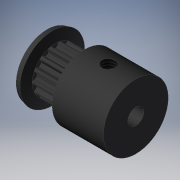
# Autodesk Inventor part: HTPB14S2M040-K-P3_a
Saved by Autodesk Inventor 2019 (Build 230136000, 136)
## iProperties
Created: 2023-12-23
Part Number: HTPB14S2M040-K-P3_a
Material: Generic
Catalog Web Link: www.cadenas.de
Description: HTPA_ _S2M040, HTPA_ _S2M060, HTPA_ _S2M100, HTPB_ _S2M040, HTPB_ _S2M060, HTPB_ _S2M100, HTPK_ _S2M040, HTPK_ _S2M060, HTPK_ _S2M100, HTPN_ _S2M040, HTPN_ _S2M060, HTPN_ _S2M100, HTPT_ _S2M040, HTPT_ _S2M060, HTPM_ _S2M040, HTPM_ _S2M060, HTPP_ _S2M040, HTPP_ _S2M060, HTPS_ _S2M040, HTPS_ _S2M060, HTPS_ _S2M100_a-High Torque Timing Pulleys S2M Type
Vendor: MISUMI
Document SubType Name: Modeling
Designer: psAdmin
Manufacturer: MISUMI
Mass: 1.31576 g
Surface Area: 11.5527 cm^2
Volume: 1.31576 cm^3
Density: 1 g/cm^3
Appearance: PSOLRGB-175-175-175
Category: PARTsolutions
Company: MISUMI
Title: HTPB14S2M040-K-P3
Author: Cadenas PARTsolutions
Comments: High Torque Timing Pulleys S2M Type
PSOL_IDENT_0: {$CADENAS_DATA/23d-libs/misumi/metric/51_timing_pulleys/htpm_s2m/htpa_s2m.prj},734 {VTYP=3D},{NB=HTP
PSOL_IDENT_1: B14S2M040-K-P3_a},{LINA=HTPB14S2M040-K-P3},{NN=HTPA_ _S2M040, HTPA_ _S2M060, HTPA_ _S2M100, HTPB_ _S
PSOL_IDENT_2: 2M040, HTPB_ _S2M060, HTPB_ _S2M100, HTPK_ _S2M040, HTPK_ _S2M060, HTPK_ _S2M100, HTPN_ _S2M040, HTP
PSOL_IDENT_3: N_ _S2M060, HTPN_ _S2M100, HTPT_ _S2M040, HTPT_ _S2M060, HTPM_ _S2M040, HTPM_ _S2M060, HTPP_ _S2M040
PSOL_IDENT_4: , HTPP_ _S2M060, HTPS_ _S2M040, HTPS_ _S2M060, HTPS_ _S2M100_a},{DATE=29.05.2023 09:16:33},{GEOMDATE=
PSOL_IDENT_5: 11.01.2023 01:57:31},{VERSION=},{LINEID=10},{WBVAR=MATP,ST,TNW,PS,SBS,DD,Z,J,Q,R,S,T,ALT1,ALT2,M,QSC
PSOL_IDENT_6: ,QFC,QTC,ALT3,K,KSC,KFC,KTC,ALT4,ZM,ZSC,ZFC,ZTC,ALT5,ALT6,ALT7,FC,ALT8,SRG,ALT9,BTC,TL,ALT10,TPC,ALT
PSOL_IDENT_7: 11,BC,ALT12,SLH,ALT13,BN},{WBNUMERIC=DD,Z,J,Q,R,S,T,QSC,QFC,QTC,K,KSC,KFC,KTC,ZSC,ZFC,ZTC,FC,SRG,BTC
PSOL_IDENT_8: ,TL,BC,SLH,BN}  {NB=HTPB14S2M040-K-P3_a},{LINA=HTPB14S2M040-K-P3},{KT=DUMMY},{PN=HTPB14S2M040-K-P3},
PSOL_IDENT_9: {TYPE=HTPB},{MATP=A2017},{MATPALG= 'A2017','Aluminum Alloy 2000 series','S45CE','1045 Carbon Steel E
PSOL_IDENT_10: quivalent','SUS304','304 Stainless Steel' },{ST=BA},{STALG= 'CA' , 'Clear Anodize', 'BA','Black Anod
PSOL_IDENT_11: ize','HAT','Hard Clear Anodize' , 'ENP' , 'Electroless Nickel Plating' },{NT=14},{TNW=S2M040},{TNWAL
PSOL_IDENT_12: G= 'S2M040', 'S2M060','S2M100' },{BW=4},{PS=K},{PSALG='A','K'},{SBS=P},{SBSALG='H','Round Hole','P','
PSOL_IDENT_13: Round Hole + Tap'},{SHSA= 'H','Round Hole' },{SHSB='H','Round Hole','P','Round Hole + Tap','N','New
PSOL_IDENT_14: JIS Keywayed Bore + Tap (Standard)','NK','New JIS Keywayed Bore + Tap (width 4.0mm, height 1.8mm)','
PSOL_IDENT_15: C','Old JIS Keywayed Bore + Tap','V','Stepped Hole','F','Stepped Hole (Counterbore holes on the boss
PSOL_IDENT_16: side)' },{SHSK='H','Round Hole','P','Round Hole + Tap'},{SBSPN=-P3},{DD=3.00},{DDALG=[3:4/1]},{DDHA=
PSOL_IDENT_17: 0},{DDHBK=[3:4/1]},{DDPA=0},{DDPBK=[3:4/1]},{DDNA=0},{DDNBK=0},{DDNK=0},{DDCA=0},{DDCBK=0},{DDVA=0},
PSOL_IDENT_18: {DDVF=0},{DDY=0},{DDWB=0},{Z=0},{ZALG=[0]},{ZQRMIN=5},{ZAMAX=0},{ZBMAX=0},{DDZ=3},{J=0.0},{JALG=[0]}
PSOL_IDENT_19: ,{JMAX=0},{JMIN=2},{JPN=},{QRMAX=0},{QRMIN=5},{WBRMAX=-2.00},{WBQMIN=7},{Q=0},{QALG=[0]},{QPN=},{R=0
PSOL_IDENT_20: },{RALG=[0]},{S=0.0},{SALG=[0]},{SPN=},{SMAX=3},{T=0.0},{TALG=[0]},{TPN=},{TMAX=6},{A=5},{W=9},{L=17
PSOL_IDENT_21: },{PD=8.91},{OD=8.40},{D=12},{DALG=12},{DE=12},{F=12},{E=6},{BBK=0.000},{TTK=0.0},{TT=1},{WL=17.000}
PSOL_IDENT_22: ,{ALT1=},{ALT1ALG= '','w/o KC90 (Set Screw Angle)','KC90','with KC90 (Set Screw Angle)' },{ANG=120.0
PSOL_IDENT_23: 00},{ALT1PN=},{ALT2=},{ALT2ALG= '','Not applicable' },{M=N/A},{MALG= 'N/A' },{MFTALG= 'N/A' },{MSALG=
PSOL_IDENT_24: 'N/A' },{M3D=0.000},{KDML=0},{ML=0},{MUL=0},{PITCH=0},{QSC=0.0},{QSCALG=0},{QFC=0.0},{QFCALG=0},{QT
PSOL_IDENT_25: C=0.0},{QTCALG=0},{QPCDMIN=0},{QPCDMINALG=0},{QPCDMAX=8},{ALT2PN=},{ALT3=},{ALT3ALG= '','Not applica
PSOL_IDENT_26: ble' },{K=0.0},{KALG=0},{KMIN=4},{KFTMAX=0.0},{KSMAX=0.0},{KSC=0.0},{KSCALG=0},{KFC=0.0},{KFCALG=0},
PSOL_IDENT_27: {KTC=0.0},{KTCALG=0},{KPCDMIN=7},{KPCDMINALG=7},{KPCDMAX=0},{KSCMIN=7.0},{KSCMINALG=7},{ALT3PN=},{AL
PSOL_IDENT_28: T4=},{ALT4ALG= '','Not applicable' },{ALT4MIN=13.5},{ALT4MAX=-4.5},{ZM=N/A},{ZMALG= 'N/A' },{ZMSALG=
PSOL_IDENT_29: 'N/A' },{ZMFTALG= 'N/A' },{ZMDD1=0.0},{ZMDD2=0.0},{ZMHH=0.0},{ZSC=0.0},{ZSCALG=[0]},{ZFC=0.0},{ZFCA
PSOL_IDENT_30: LG=[0]},{ZTC=0.0},{ZTCALG=[0]},{ZPCDMIN=0},{ZPCDMINALG=0},{ZPCDMAX=2},{ALT4PN=},{ALT5=},{ALT5ALG= ''
PSOL_IDENT_31: ,'Flange Attached','NFC','with NFC (Flange not Attached)' },{ALT5PN=},{ALT6=},{ALT6ALG= '','Not appl
PSOL_IDENT_32: icable' },{ALT6PN=},{ALT7=},{ALT7ALG= '','w/o FC (Flange Cut)','FC','with FC (Flange Cut)' },{FC=0.0
PSOL_IDENT_33: },{FCALG=0},{FCMIN=9.5},{FCMAX=10.0},{ALT7PN=},{ALT8=},{ALT8ALG= '','Not applicable' },{ALT8ALGALG=8
PSOL_IDENT_34: },{ALT8DD2=0},{ALT8MM=0},{ALT8NN=0},{QC=0},{KC=0},{ZC=0},{SRG=0.0},{SRGALG=[0]},{SRGMAX=0},{DD2=0.0}
PSOL_IDENT_35: ,{MM=0.00},{NN=0.00},{ALT8PN=},{ALT9ALG= '','Not applicable' },{ALT9=},{BTC9=4},{TL9=1},{BTC=0},{BTC
PSOL_IDENT_36: ALG=[0]},{TL=0.0},{TLALG=[0]},{TLMIN=1.0},{TLMAX=-9.5},{BTCL=0},{BTCD=0},{BTCDALG=6.000},{ALT9PN=},{
PSOL_IDENT_37: WLBCTL=17},{ALT10=},{ALT10ALG= '','w/o TPC (Tapped Hole Dimension)','TPC','with TPC (Tapped Hole Dim
PSOL_IDENT_38: ension)' },{TPC=N/A},{TPCALG= 'N/A' },{TPCM=3},{ALT10PN=},{ALT11=},{ALT11ALG= '','Not applicable' },
PSOL_IDENT_39: {BC=0.0},{BCALG=0},{BCMIN=6},{BCMAX=7.5},{BCPLANE=12},{M1WBC=12},{ALT11PN=},{ALT12=},{ALT12ALG= '','
PSOL_IDENT_40: w/o SLH (Set Screw Length)','SLH','with SLH (Set Screw Length)' },{SLH=0},{SLHALG=[0]},{ALT12PN=},{A
PSOL_IDENT_41: LT13=},{ALT13ALG= '', 'Not applicable' },{BN=0.0},{BNALG=0},{BNMIN=8.5},{BNMAX=18},{ALT13PN=},{AC=M3
PSOL_IDENT_42: x3},{M1=3},{M1L=3},{TAP=0.000},{KYY=1.5},{KTT=4.5},{PLANE=0},{CD=9},{SRGCUT=1}
NB: HTPB14S2M040-K-P3_a
NN: HTPA_ _S2M040, HTPA_ _S2M060, HTPA_ _S2M100, HTPB_ _S2M040, HTPB_ _S2M060, HTPB_ _S2M100, HTPK_ _S2M040, HTPK_ _S2M060, HTPK_ _S2M100, HTPN_ _S2M040, HTPN_ _S2M060, HTPN_ _S2M100, HTPT_ _S2M040, HTPT_ _S2M060, HTPM_ _S2M040, HTPM_ _S2M060, HTPP_ _S2M040, HTPP_ _S2M060, HTPS_ _S2M040, HTPS_ _S2M060, HTPS_ _S2M100_a
NT: 14
NBSYN: $PN._a
LINA: HTPB14S2M040-K-P3
CATALOG: Misumi
PN: HTPB14S2M040-K-P3
MATP: Aluminum Alloy 2000 series
ST: Black Anodize
TNW: S2M040
BW: 4
PS: K
SBS: Round Hole + Tap
DD: 3
Z: 0
J: 0
Q: 0
R: 0
S: 0
T: 0
A: 5
W: 9
L: 17
PD: 8.91
OD: 8.4
D: 12
F: 12
ALT1: w/o KC90 (Set Screw Angle)
ALT2: Not applicable
M: N/A
QSC: 0
QFC: 0
QTC: 0
ALT3: Not applicable
K: 0
KSC: 0
KFC: 0
KTC: 0
ALT4: Not applicable
ZM: N/A
ZSC: 0
ZFC: 0
ZTC: 0
ALT5: Flange Attached
ALT6: Not applicable
ALT7: w/o FC (Flange Cut)
FC: 0
ALT8: Not applicable
SRG: 0
ALT9: Not applicable
BTC: 0
TL: 0
ALT10: w/o TPC (Tapped Hole Dimension)
TPC: N/A
ALT11: Not applicable
BC: 0
ALT12: w/o SLH (Set Screw Length)
SLH: 0
ALT13: Not applicable
BN: 0
AC: M3x3
SUPPLIER: MISUMI
ARTICLENO: HTPB14S2M040-K-P3_a
BOMINFO: HTPB14S2M040-K-P3
CREATOR: CADENAS GmbH
Autodesk Inventor part; units mm, degrees
sketch "_____3" plane through (0, 0, 0) normal (0, 0, 1) x (1, 0, 0)
  line L0 (17, 0) -> (0, 0)
  line L1 (0, 0) -> (0, 3)
  line L2 (0, 3) -> (1, 3)
  line L3 (1, 3) -> (1, 4.068348)
  line L4 (1, 4.068348) -> (0.551766, 5.741181)
  line L5 (0.551766, 5.741181) -> (1.517691, 6)
  line L6 (1.517691, 6) -> (2, 4.2)
  line L7 (2, 4.2) -> (7, 4.2)
  line L8 (7, 4.2) -> (7, 4.5)
  line L9 (7, 4.5) -> (7.5, 6)
  line L10 (7.5, 6) -> (17, 6)
  line L11 (17, 6) -> (17, 0)
  line L12 (17, 0) -> (0, 0)
  constraints: 26 end point
revolve "Revolution1" add sketch "_____3" angle 360 about axis through (17, 0, 0) along (1, 0, 0)
sketch "Sketch2" plane through (17, 0, 0) normal (1, 0, 0) x (0, 0, -1)
  point P0 (0, 0)
hole "Hole1" at (17, 0, 0) direction (-1, 0, 0) diameter 3 depth 17
sketch "_____6" plane through (2, 0, 0) normal (1, 0, 0) x (0, 0, -1)
  circle A0 centre (0, 0) radius 8.4
  arc A1 (-4.2, 0) -> (-4.198526, -0.11128) centre (0, 0) ccw
  arc A2 (-4.198526, -0.11128) -> (-4.026601, -0.295391) centre (-4.008592, -0.106246) ccw
  arc A3 (-3.437791, -0.498512) -> (-4.026601, -0.295391) centre (-4.152187, -1.614426) ccw
  arc A4 (-3.393072, -0.56627) -> (-3.437791, -0.498512) centre (-3.491708, -0.582731) ccw
  arc A5 (-3.393072, -0.56627) -> (-3.302748, -0.962007) centre (0, 0) ccw
  arc A6 (-3.313639, -1.042458) -> (-3.302748, -0.962007) centre (-3.398758, -0.989972) ccw
  arc A7 (-3.756007, -1.480939) -> (-3.313639, -1.042458) centre (-4.441464, -0.347019) ccw
  arc A8 (-3.756007, -1.480939) -> (-3.831023, -1.721412) centre (-3.657715, -1.643539) ccw
  arc A9 (-3.831023, -1.721412) -> (-3.784069, -1.822312) centre (0, 0) ccw
  arc A10 (-3.784069, -1.822312) -> (-3.734458, -1.921932) centre (0, 0) ccw
  arc A11 (-3.734458, -1.921932) -> (-3.499677, -2.013214) centre (-3.565518, -1.834987) ccw
  arc A12 (-2.881047, -1.940745) -> (-3.499677, -2.013214) centre (-3.040518, -3.256113) ccw
  arc A13 (-2.811357, -1.982391) -> (-2.881047, -1.940745) centre (-2.893082, -2.040018) ccw
  arc A14 (-2.811357, -1.982391) -> (-2.558274, -2.299747) centre (0, 0) ccw
  arc A15 (-2.53318, -2.376957) -> (-2.558274, -2.299747) centre (-2.632642, -2.3666) ccw
  arc A16 (-2.74149, -2.96395) -> (-2.53318, -2.376957) centre (-3.851055, -2.239733) ccw
  arc A17 (-2.74149, -2.96395) -> (-2.70474, -3.213157) centre (-2.582383, -3.0678) ccw
  arc A18 (-2.70474, -3.213157) -> (-2.618657, -3.283692) centre (0, 0) ccw
  arc A19 (-2.618657, -3.283692) -> (-2.530736, -3.351921) centre (0, 0) ccw
  arc A20 (-2.530736, -3.351921) -> (-2.279599, -3.332296) centre (-2.41625, -3.200287) ccw
  arc A21 (-1.753676, -2.99859) -> (-2.279599, -3.332296) centre (-1.326637, -4.252888) ccw
  arc A22 (-1.672818, -3.005874) -> (-1.753676, -2.99859) centre (-1.721446, -3.093254) ccw
  arc A23 (-1.672818, -3.005874) -> (-1.307102, -3.181994) centre (0, 0) ccw
  arc A24 (-1.250993, -3.240669) -> (-1.307102, -3.181994) centre (-1.345099, -3.274494) ccw
  arc A25 (-1.183987, -3.859915) -> (-1.250993, -3.240669) centre (-2.497897, -3.688839) ccw
  arc A26 (-1.183987, -3.859915) -> (-1.04275, -4.068498) centre (-0.995578, -3.884447) ccw
  arc A27 (-1.04275, -4.068498) -> (-0.934588, -4.094697) centre (0, 0) ccw
  arc A28 (-0.934588, -4.094697) -> (-0.82577, -4.118022) centre (0, 0) ccw
  arc A29 (-0.82577, -4.118022) -> (-0.608018, -3.991376) centre (-0.788414, -3.93173) ccw
  arc A30 (-0.278968, -3.462528) -> (-0.608018, -3.991376) centre (0.65, -4.407326) ccw
  arc A31 (-0.202957, -3.434008) -> (-0.278968, -3.462528) centre (-0.208857, -3.533833) ccw
  arc A32 (-0.202957, -3.434008) -> (0.202957, -3.434008) centre (0, 0) ccw
  arc A33 (0.278968, -3.462528) -> (0.202957, -3.434008) centre (0.208857, -3.533833) ccw
  arc A34 (0.608018, -3.991376) -> (0.278968, -3.462528) centre (-0.65, -4.407326) ccw
  arc A35 (0.608018, -3.991376) -> (0.82577, -4.118022) centre (0.788414, -3.93173) ccw
  arc A36 (0.82577, -4.118022) -> (0.934588, -4.094697) centre (0, 0) ccw
  arc A37 (0.934588, -4.094697) -> (1.04275, -4.068498) centre (0, 0) ccw
  arc A38 (1.04275, -4.068498) -> (1.183987, -3.859915) centre (0.995578, -3.884447) ccw
  arc A39 (1.250993, -3.240669) -> (1.183987, -3.859915) centre (2.497897, -3.688839) ccw
  arc A40 (1.307102, -3.181994) -> (1.250993, -3.240669) centre (1.345099, -3.274494) ccw
  arc A41 (1.307102, -3.181994) -> (1.672818, -3.005874) centre (0, 0) ccw
  arc A42 (1.753676, -2.99859) -> (1.672818, -3.005874) centre (1.721446, -3.093254) ccw
  arc A43 (2.279599, -3.332296) -> (1.753676, -2.99859) centre (1.326637, -4.252888) ccw
  arc A44 (2.279599, -3.332296) -> (2.530736, -3.351921) centre (2.41625, -3.200287) ccw
  arc A45 (2.530736, -3.351921) -> (2.618657, -3.283692) centre (0, 0) ccw
  arc A46 (2.618657, -3.283692) -> (2.70474, -3.213157) centre (0, 0) ccw
  arc A47 (2.70474, -3.213157) -> (2.74149, -2.96395) centre (2.582383, -3.0678) ccw
  arc A48 (2.53318, -2.376957) -> (2.74149, -2.96395) centre (3.851055, -2.239733) ccw
  arc A49 (2.558274, -2.299747) -> (2.53318, -2.376957) centre (2.632642, -2.3666) ccw
  arc A50 (2.558274, -2.299747) -> (2.811357, -1.982391) centre (0, 0) ccw
  arc A51 (2.881047, -1.940745) -> (2.811357, -1.982391) centre (2.893082, -2.040018) ccw
  arc A52 (3.499677, -2.013214) -> (2.881047, -1.940745) centre (3.040518, -3.256113) ccw
  arc A53 (3.499677, -2.013214) -> (3.734458, -1.921932) centre (3.565518, -1.834987) ccw
  arc A54 (3.734458, -1.921932) -> (3.784069, -1.822312) centre (0, 0) ccw
  arc A55 (3.784069, -1.822312) -> (3.831023, -1.721412) centre (0, 0) ccw
  arc A56 (3.831023, -1.721412) -> (3.756007, -1.480939) centre (3.657715, -1.643539) ccw
  arc A57 (3.313639, -1.042458) -> (3.756007, -1.480939) centre (4.441464, -0.347019) ccw
  arc A58 (3.302748, -0.962007) -> (3.313639, -1.042458) centre (3.398758, -0.989972) ccw
  arc A59 (3.302748, -0.962007) -> (3.393072, -0.56627) centre (0, 0) ccw
  arc A60 (3.437791, -0.498512) -> (3.393072, -0.56627) centre (3.491708, -0.582731) ccw
  arc A61 (4.026601, -0.295391) -> (3.437791, -0.498512) centre (4.152187, -1.614426) ccw
  arc A62 (4.026601, -0.295391) -> (4.198526, -0.11128) centre (4.008592, -0.106246) ccw
  arc A63 (4.198526, -0.11128) -> (4.2, 0) centre (0, 0) ccw
  arc A64 (4.2, 0) -> (4.198526, 0.11128) centre (0, 0) ccw
  arc A65 (4.198526, 0.11128) -> (4.026601, 0.295391) centre (4.008592, 0.106246) ccw
  arc A66 (3.437791, 0.498512) -> (4.026601, 0.295391) centre (4.152187, 1.614426) ccw
  arc A67 (3.393072, 0.56627) -> (3.437791, 0.498512) centre (3.491708, 0.582731) ccw
  arc A68 (3.393072, 0.56627) -> (3.302748, 0.962007) centre (0, 0) ccw
  arc A69 (3.313639, 1.042458) -> (3.302748, 0.962007) centre (3.398758, 0.989972) ccw
  arc A70 (3.756007, 1.480939) -> (3.313639, 1.042458) centre (4.441464, 0.347019) ccw
  arc A71 (3.756007, 1.480939) -> (3.831023, 1.721412) centre (3.657715, 1.643539) ccw
  arc A72 (3.831023, 1.721412) -> (3.784069, 1.822312) centre (0, 0) ccw
  arc A73 (3.784069, 1.822312) -> (3.734458, 1.921932) centre (0, 0) ccw
  arc A74 (3.734458, 1.921932) -> (3.499677, 2.013214) centre (3.565518, 1.834987) ccw
  arc A75 (2.881047, 1.940745) -> (3.499677, 2.013214) centre (3.040518, 3.256113) ccw
  arc A76 (2.811357, 1.982391) -> (2.881047, 1.940745) centre (2.893082, 2.040018) ccw
  arc A77 (2.811357, 1.982391) -> (2.558274, 2.299747) centre (0, 0) ccw
  arc A78 (2.53318, 2.376957) -> (2.558274, 2.299747) centre (2.632642, 2.3666) ccw
  arc A79 (2.74149, 2.96395) -> (2.53318, 2.376957) centre (3.851055, 2.239733) ccw
  arc A80 (2.74149, 2.96395) -> (2.70474, 3.213157) centre (2.582383, 3.0678) ccw
  arc A81 (2.70474, 3.213157) -> (2.618657, 3.283692) centre (0, 0) ccw
  arc A82 (2.618657, 3.283692) -> (2.530736, 3.351921) centre (0, 0) ccw
  arc A83 (2.530736, 3.351921) -> (2.279599, 3.332296) centre (2.41625, 3.200287) ccw
  arc A84 (1.753676, 2.99859) -> (2.279599, 3.332296) centre (1.326637, 4.252888) ccw
  arc A85 (1.672818, 3.005874) -> (1.753676, 2.99859) centre (1.721446, 3.093254) ccw
  arc A86 (1.672818, 3.005874) -> (1.307102, 3.181994) centre (0, 0) ccw
  arc A87 (1.250993, 3.240669) -> (1.307102, 3.181994) centre (1.345099, 3.274494) ccw
  arc A88 (1.183987, 3.859915) -> (1.250993, 3.240669) centre (2.497897, 3.688839) ccw
  arc A89 (1.183987, 3.859915) -> (1.04275, 4.068498) centre (0.995578, 3.884447) ccw
  arc A90 (1.04275, 4.068498) -> (0.934588, 4.094697) centre (0, 0) ccw
  arc A91 (0.934588, 4.094697) -> (0.82577, 4.118022) centre (0, 0) ccw
  arc A92 (0.82577, 4.118022) -> (0.608018, 3.991376) centre (0.788414, 3.93173) ccw
  arc A93 (0.278968, 3.462528) -> (0.608018, 3.991376) centre (-0.65, 4.407326) ccw
  arc A94 (0.202957, 3.434008) -> (0.278968, 3.462528) centre (0.208857, 3.533833) ccw
  arc A95 (0.202957, 3.434008) -> (-0.202957, 3.434008) centre (0, 0) ccw
  arc A96 (-0.278968, 3.462528) -> (-0.202957, 3.434008) centre (-0.208857, 3.533833) ccw
  arc A97 (-0.608018, 3.991376) -> (-0.278968, 3.462528) centre (0.65, 4.407326) ccw
  arc A98 (-0.608018, 3.991376) -> (-0.82577, 4.118022) centre (-0.788414, 3.93173) ccw
  arc A99 (-0.82577, 4.118022) -> (-0.934588, 4.094697) centre (0, 0) ccw
  arc A100 (-0.934588, 4.094697) -> (-1.04275, 4.068498) centre (0, 0) ccw
  arc A101 (-1.04275, 4.068498) -> (-1.183987, 3.859915) centre (-0.995578, 3.884447) ccw
  arc A102 (-1.250993, 3.240669) -> (-1.183987, 3.859915) centre (-2.497897, 3.688839) ccw
  arc A103 (-1.307102, 3.181994) -> (-1.250993, 3.240669) centre (-1.345099, 3.274494) ccw
  arc A104 (-1.307102, 3.181994) -> (-1.672818, 3.005874) centre (0, 0) ccw
  arc A105 (-1.753676, 2.99859) -> (-1.672818, 3.005874) centre (-1.721446, 3.093254) ccw
  arc A106 (-2.279599, 3.332296) -> (-1.753676, 2.99859) centre (-1.326637, 4.252888) ccw
  arc A107 (-2.279599, 3.332296) -> (-2.530736, 3.351921) centre (-2.41625, 3.200287) ccw
  arc A108 (-2.530736, 3.351921) -> (-2.618657, 3.283692) centre (0, 0) ccw
  arc A109 (-2.618657, 3.283692) -> (-2.70474, 3.213157) centre (0, 0) ccw
  arc A110 (-2.70474, 3.213157) -> (-2.74149, 2.96395) centre (-2.582383, 3.0678) ccw
  arc A111 (-2.53318, 2.376957) -> (-2.74149, 2.96395) centre (-3.851055, 2.239733) ccw
  arc A112 (-2.558274, 2.299747) -> (-2.53318, 2.376957) centre (-2.632642, 2.3666) ccw
  arc A113 (-2.558274, 2.299747) -> (-2.811357, 1.982391) centre (0, 0) ccw
  arc A114 (-2.881047, 1.940745) -> (-2.811357, 1.982391) centre (-2.893082, 2.040018) ccw
  arc A115 (-3.499677, 2.013214) -> (-2.881047, 1.940745) centre (-3.040518, 3.256113) ccw
  arc A116 (-3.499677, 2.013214) -> (-3.734458, 1.921932) centre (-3.565518, 1.834987) ccw
  arc A117 (-3.734458, 1.921932) -> (-3.784069, 1.822312) centre (0, 0) ccw
  arc A118 (-3.784069, 1.822312) -> (-3.831023, 1.721412) centre (0, 0) ccw
  arc A119 (-3.831023, 1.721412) -> (-3.756007, 1.480939) centre (-3.657715, 1.643539) ccw
  arc A120 (-3.313639, 1.042458) -> (-3.756007, 1.480939) centre (-4.441464, 0.347019) ccw
  arc A121 (-3.302748, 0.962007) -> (-3.313639, 1.042458) centre (-3.398758, 0.989972) ccw
  arc A122 (-3.302748, 0.962007) -> (-3.393072, 0.56627) centre (0, 0) ccw
  arc A123 (-3.437791, 0.498512) -> (-3.393072, 0.56627) centre (-3.491708, 0.582731) ccw
  arc A124 (-4.026601, 0.295391) -> (-3.437791, 0.498512) centre (-4.152187, 1.614426) ccw
  arc A125 (-4.026601, 0.295391) -> (-4.198526, 0.11128) centre (-4.008592, 0.106246) ccw
  arc A126 (-4.198526, 0.11128) -> (-4.2, 0) centre (0, 0) ccw
  constraints: 252 point on circle, 127 centre point
extrude "Extrusion1" cut sketch "_____6" along normal blind 5
sketch "_____20" plane through (12, 0, 0) normal (1, 0, 0) x (0, 0, -1)
  line L0 (0, 0) -> (0, 6)
  line L1 (0, 6) -> (1.2295, 6)
  line L2 (1.2295, 6) -> (1.2295, 0)
  line L3 (1.2295, 0) -> (0, 0)
  line L4 (0, 0) -> (0, 6)
  constraints: 10 end point
revolve "Revolution2" cut sketch "_____20" angle 360 about axis through (12, 0, 0) along (0, -1, 0)
thread "Thread1" size "M3x0.5" class "6H" standard "ISO Metric profile" length 4.5
sketch "_____21" plane through (12, 0, 0) normal (1, 0, 0) x (0, 0, -1)
  line L0 (0, 0) -> (5.196152, -3)
  line L1 (5.196152, -3) -> (4.581402, -4.064778)
  line L2 (4.581402, -4.064778) -> (-0.61475, -1.064778)
  line L3 (-0.61475, -1.064778) -> (0, 0)
  line L4 (0, 0) -> (5.196152, -3)
  constraints: 10 end point
revolve "Revolution3" cut sketch "_____21" angle 360 about axis through (12, 0, 0) along (0, 0.5, 0.8660254)
thread "Thread2" size "M3x0.5" class "6H" standard "ISO Metric profile" length 4.5
ref_plane "C1_XY" through (4.5, 0, 0) normal (1, 0, 0) x (0, 0, -1)
ref_plane "C1_YZ" through (4.5, 0, 0) normal (0, 0, -1) x (0, 1, 0)
ref_plane "C1_ZX" through (4.5, 0, 0) normal (0, 1, 0) x (1, 0, 0)
ref_plane "to_belt_XY" through (4.5, 0, 0) normal (-1, 0, 0) x (0, 0, -1)
ref_plane "to_belt_YZ" through (4.5, 0, 0) normal (0, 0, -1) x (0, -1, 0)
ref_plane "to_belt_ZX" through (4.5, 0, 0) normal (0, -1, 0) x (-1, 0, 0)
ref_plane "to_s1_XY" through (12, 1.5, 0) normal (0, 1, 0) x (1, 0, 0)
ref_plane "to_s1_YZ" through (12, 1.5, 0) normal (1, 0, 0) x (0, 0, -1)
ref_plane "to_s1_ZX" through (12, 1.5, 0) normal (0, 0, -1) x (0, 1, 0)
ref_plane "to_s2_XY" through (12, -0.75, -1.299038) normal (0, -0.5, -0.8660254) x (1, 0, 0)
ref_plane "to_s2_YZ" through (12, -0.75, -1.299038) normal (1, 0, 0) x (0, -0.8660254, 0.5)
ref_plane "to_s2_ZX" through (12, -0.75, -1.299038) normal (0, -0.8660254, 0.5) x (0, -0.5, -0.8660254)
body "Solid1"
